Autodesk Inventor part; units mm, degrees
(part 2 of 2)
sketch "Skizze22" plane through (45, 45.75, 168) normal (0, 1, 0) x (1, 0, 0)
  line L0 (15, 0) -> (0, 0) projected
  line L1 (15, 168) -> (15, 0) projected
  line L2 (0, 168) -> (15, 168) projected
  line L3 (-105, 0) -> (-105, 168) projected
  line L4 (-105, 168) -> (-90, 168) projected
  line L5 (-90, 0) -> (-105, 0) projected
  circle A0 centre (-97.5, 7.5) radius 1.35 projected
  circle A1 centre (-97.5, 7.5) radius 1.7
  circle A2 centre (7.5, 7.5) radius 1.7
  circle A3 centre (7.5, 142.5) radius 1.7
  circle A4 centre (-97.5, 142.5) radius 1.7
  circle A5 centre (-97.5, 7.5) radius 1.35 construction
  line L6 (-97.5, 7.5) -> (-97.5, 142.5) construction
  line L7 (7.5, 142.5) -> (7.5, 7.5) construction
  circle A6 centre (7.5, 57.5) radius 1.7
  circle A7 centre (-97.5, 57.5) radius 1.7
  circle A8 centre (112.5, -130.5) radius 1.35
  circle A9 centre (112.5, -130.5) radius 1.7
  circle A10 centre (7.5, -130.5) radius 1.35
  circle A11 centre (7.5, -130.5) radius 1.7
  circle A12 centre (7.5, -25.5) radius 1.35
  circle A13 centre (7.5, -25.5) radius 1.7
  circle A14 centre (112.5, -25.5) radius 1.35
  circle A15 centre (112.5, -25.5) radius 1.7
  circle A16 centre (7.5, 7.5) radius 1.35
  circle A17 centre (7.5, 7.5) radius 1.7
  circle A18 centre (-97.5, 7.5) radius 1.35
  circle A19 centre (-97.5, 7.5) radius 1.7
  circle A20 centre (-97.5, 112.5) radius 1.35
  circle A21 centre (-97.5, 112.5) radius 1.7
  circle A22 centre (7.5, 112.5) radius 1.35
  circle A23 centre (7.5, 112.5) radius 1.7
  point P0 (-45, 168)
  point P1 (-97.5, 142.5)
  point P2 (-98.85, 7.5)
  point P3 (-98.85, 7.5)
  point P4 (7.5, 57.5)
  point P5 (60, 0)
  dimension "d104" = 7.5
  dimension "d105" = 7.5
  dimension "d106" = 25.5
  dimension "d107" = 7.5
  dimension "d108" = 7.5
  dimension "d109" = 25.5
  dimension "d110" = 7.5
  dimension "d111" = 7.5
  dimension "d113" = 3.4
  dimension "d114" = 3.4
  dimension "d115" = 3.4
  dimension "d129" = 3.4
  dimension "d130" = 135
  dimension "d131" = 50
  dimension "d132" = 50
  dimension "d133" = 3.4
  dimension "d134" = 3.4
  dimension "d165" = 3.4
  dimension "d166" = 3.4
  dimension "d167" = 3.4
  dimension "d168" = 3.4
  dimension "d169" = 3.4
  dimension "d170" = 3.4
  dimension "d171" = 3.4
  dimension "d172" = 3.4
  constraints: 22 centre point, 11 coincident, 4 end point, 2 point on line, 1 parallel
  measures "d104" distance from line of L0 point (7.5, 7.5)
  measures "d105" distance from line of L1 point (7.5, 7.5)
  measures "d106" distance from line of L2 point (7.5, 142.5)
  measures "d107" distance from line of L1 point (7.5, 142.5)
  measures "d108" distance from line of L3 point (-97.5, 142.5)
  measures "d109" distance from line of L4 point (-97.5, 142.5)
  measures "d110" distance from line of L3 point (-97.5, 7.5)
  measures "d111" distance from line of L5 point (-97.5, 7.5)
  measures "d113" diameter of A3
  measures "d114" diameter of A2
  measures "d115" diameter of A1
  measures "d129" diameter of A4
  measures "d130" distance of L7.start L7.end
  measures "d131" distance of point (7.5, 7.5) point (7.5, 57.5)
  measures "d132" distance of point (-97.5, 7.5) point (-97.5, 57.5)
  measures "d133" diameter of A6
  measures "d134" diameter of A7
  measures "d165" diameter of A15
  measures "d166" diameter of A13
  measures "d167" diameter of A11
  measures "d168" diameter of A9
  measures "d169" diameter of A23
  measures "d170" diameter of A21
  measures "d171" diameter of A19
  measures "d172" diameter of A17
extrude "Extrusion15" cut sketch "Skizze22" against normal blind 60 contours A0 | A1 | A2 | A3 | A4 | A6 | A7 | A16 | A20 | A21 | A22 | A23
ref_plane "Arbeitsebene1" through (45, 35.75, 168) normal (0, 1, 0) x (1, 0, 0)
sketch "Skizze23" plane through (45, 35.75, 168) normal (0, 1, 0) x (1, 0, 0)
  circle A0 centre (7.5, 7.5) radius 1.7 projected
  line L0 (4.65, 9.1454) -> (7.5, 10.7909)
  line L1 (7.5, 10.7909) -> (10.35, 9.1454)
  line L2 (10.35, 9.1454) -> (10.35, 5.8546)
  line L3 (10.35, 5.8546) -> (7.5, 4.2091)
  line L4 (7.5, 4.2091) -> (4.65, 5.8546)
  line L5 (4.65, 5.8546) -> (4.65, 9.1454)
  line L6 (0, 149.5) -> (0, 0) projected
  circle A1 centre (-97.5, 7.5) radius 1.7 projected
  circle A2 centre (7.5, 142.5) radius 1.7 projected
  line L7 (-100.35, 9.1454) -> (-97.5, 10.7909)
  line L8 (-97.5, 10.7909) -> (-94.65, 9.1454)
  line L9 (-94.65, 9.1454) -> (-94.65, 5.8546)
  line L10 (-94.65, 5.8546) -> (-97.5, 4.2091)
  line L11 (-97.5, 4.2091) -> (-100.35, 5.8546)
  line L12 (-100.35, 5.8546) -> (-100.35, 9.1454)
  line L13 (15, 0) -> (0, 0)
  line L14 (15, 168) -> (15, 0)
  line L15 (0, 168) -> (15, 168)
  line L16 (-105, 0) -> (-105, 168)
  line L17 (-105, 168) -> (-90, 168)
  line L18 (-90, 0) -> (-105, 0)
  circle A3 centre (-97.5, 7.5) radius 1.35
  circle A4 centre (-97.5, 7.5) radius 1.7
  circle A5 centre (7.5, 7.5) radius 1.7
  circle A6 centre (7.5, 142.5) radius 1.7
  circle A7 centre (-97.5, 142.5) radius 1.7
  circle A8 centre (-97.5, 7.5) radius 1.35 construction
  line L19 (7.5, 142.5) -> (7.5, 7.5) construction
  line L20 (7.5, 4.2091) -> (15, 4.2091)
  line L21 (15, 0) -> (15, 168) projected
  line L22 (7.5, 10.7909) -> (15, 10.7909)
  line L23 (15, 4.2091) -> (15, 10.7909)
  line L24 (-97.5, 4.2091) -> (-105, 4.2091)
  line L25 (-105, 168) -> (-105, 0) projected
  line L26 (-97.5, 10.7909) -> (-105, 10.7909)
  line L27 (-105, 4.2091) -> (-105, 10.7909)
  line L28 (4.65, 144.1454) -> (7.5, 145.7909)
  line L29 (7.5, 145.7909) -> (10.35, 144.1454)
  line L30 (10.35, 144.1454) -> (10.35, 140.8546)
  line L31 (10.35, 140.8546) -> (7.5, 139.2091)
  line L32 (7.5, 139.2091) -> (4.65, 140.8546)
  line L33 (4.65, 140.8546) -> (4.65, 144.1454)
  line L34 (-100.35, 140.8546) -> (-100.35, 144.1454)
  line L35 (-100.35, 144.1454) -> (-97.5, 145.7909)
  line L36 (-97.5, 145.7909) -> (-94.65, 144.1454)
  line L37 (-94.65, 144.1454) -> (-94.65, 140.8546)
  line L38 (-94.65, 140.8546) -> (-97.5, 139.2091)
  line L39 (-97.5, 139.2091) -> (-100.35, 140.8546)
  circle A9 centre (7.5, 142.5) radius 1.7
  circle A10 centre (-97.5, 142.5) radius 1.35
  circle A11 centre (-97.5, 142.5) radius 1.35 construction
  circle A12 centre (-97.5, 142.5) radius 1.7
  line L40 (7.5, 139.2091) -> (15, 139.2091)
  line L41 (7.5, 145.7909) -> (15, 145.7909)
  line L42 (15, 139.2091) -> (15, 145.7909)
  line L43 (-97.5, 139.2091) -> (-105, 139.2091)
  line L44 (-97.5, 145.7909) -> (-105, 145.7909)
  line L45 (-105, 139.2091) -> (-105, 145.7909)
  line L46 (15, 0) -> (0, 0)
  line L47 (15, 168) -> (15, 0)
  line L48 (0, 168) -> (15, 168)
  line L49 (-105, 0) -> (-105, 168)
  line L50 (-105, 168) -> (-90, 168)
  line L51 (-90, 0) -> (-105, 0)
  circle A13 centre (-97.5, 7.5) radius 1.35
  circle A14 centre (-97.5, 7.5) radius 1.7
  circle A15 centre (7.5, 7.5) radius 1.7
  circle A16 centre (7.5, 142.5) radius 1.7
  circle A17 centre (-97.5, 142.5) radius 1.7
  circle A18 centre (-97.5, 7.5) radius 1.35 construction
  line L52 (-97.5, 7.5) -> (-97.5, 142.5) construction
  line L53 (7.5, 142.5) -> (7.5, 7.5) construction
  circle A19 centre (7.5, 57.5) radius 1.7
  circle A20 centre (-97.5, 57.5) radius 1.7
  circle A21 centre (-97.5, 112.5) radius 1.35
  circle A22 centre (-97.5, 112.5) radius 1.7
  circle A23 centre (-97.5, 7.5) radius 1.35
  circle A24 centre (-97.5, 7.5) radius 1.7
  circle A25 centre (7.5, 112.5) radius 1.35
  circle A26 centre (7.5, 112.5) radius 1.7
  circle A27 centre (7.5, 7.5) radius 1.35
  circle A28 centre (7.5, 7.5) radius 1.7
  circle A29 centre (7.5, 57.5) radius 1.7
  circle A30 centre (-97.5, 57.5) radius 1.7
  line L54 (4.65, 59.1454) -> (7.5, 60.7909)
  line L55 (7.5, 60.7909) -> (10.35, 59.1454)
  line L56 (10.35, 59.1454) -> (10.35, 55.8546)
  line L57 (10.35, 55.8546) -> (7.5, 54.2091)
  line L58 (7.5, 54.2091) -> (4.65, 55.8546)
  line L59 (4.65, 55.8546) -> (4.65, 59.1454)
  circle A31 centre (7.5, 57.5) radius 1.7
  line L60 (15, 54.2091) -> (15, 60.7909)
  line L61 (7.5, 54.2091) -> (15, 54.2091)
  line L62 (-97.5, 60.7909) -> (-94.65, 59.1454)
  line L63 (-94.65, 59.1454) -> (-94.65, 55.8546)
  line L64 (-100.35, 59.1454) -> (-97.5, 60.7909)
  line L65 (-94.65, 55.8546) -> (-97.5, 54.2091)
  line L66 (-100.35, 55.8546) -> (-100.35, 59.1454)
  line L67 (-97.5, 54.2091) -> (-100.35, 55.8546)
  line L68 (7.5, 60.7909) -> (15, 60.7909)
  line L69 (-97.5, 60.7909) -> (-105, 60.7909)
  circle A32 centre (-97.5, 57.5) radius 1.35
  circle A33 centre (-97.5, 57.5) radius 1.35 construction
  circle A34 centre (-97.5, 57.5) radius 1.7
  line L70 (-105, 54.2091) -> (-105, 60.7909)
  line L71 (-97.5, 54.2091) -> (-105, 54.2091)
  circle A35 centre (7.5, 112.5) radius 1.7
  circle A36 centre (-97.5, 112.5) radius 1.7
  line L72 (4.65, 114.1454) -> (7.5, 115.7909)
  line L73 (7.5, 115.7909) -> (10.35, 114.1454)
  line L74 (10.35, 114.1454) -> (10.35, 110.8546)
  line L75 (10.35, 110.8546) -> (7.5, 109.2091)
  line L76 (7.5, 109.2091) -> (4.65, 110.8546)
  line L77 (4.65, 110.8546) -> (4.65, 114.1454)
  circle A37 centre (7.5, 112.5) radius 1.7
  line L78 (15, 109.2091) -> (15, 115.7909)
  line L79 (7.5, 109.2091) -> (15, 109.2091)
  line L80 (-97.5, 115.7909) -> (-94.65, 114.1454)
  line L81 (-94.65, 114.1454) -> (-94.65, 110.8546)
  line L82 (-100.35, 114.1454) -> (-97.5, 115.7909)
  line L83 (-94.65, 110.8546) -> (-97.5, 109.2091)
  line L84 (-100.35, 110.8546) -> (-100.35, 114.1454)
  line L85 (-97.5, 109.2091) -> (-100.35, 110.8546)
  line L86 (7.5, 115.7909) -> (15, 115.7909)
  line L87 (-97.5, 115.7909) -> (-105, 115.7909)
  circle A38 centre (-97.5, 112.5) radius 1.35
  circle A39 centre (-97.5, 112.5) radius 1.35 construction
  circle A40 centre (-97.5, 112.5) radius 1.7
  line L88 (-105, 109.2091) -> (-105, 115.7909)
  line L89 (-97.5, 109.2091) -> (-105, 109.2091)
  point P0 (-45, 168)
  point P1 (-45, 168)
  point P2 (-97.5, 142.5)
  point P3 (-98.85, 7.5)
  point P4 (-98.85, 7.5)
  point P5 (-98.85, 142.5)
  point P6 (-98.85, 142.5)
  point P7 (-105, 10.7909)
  point P8 (7.5, 4.2091)
  point P9 (15, 4.2091)
  point P10 (15, 10.7909)
  point P11 (-45, 168)
  point P12 (-97.5, 142.5)
  point P13 (-98.85, 7.5)
  point P14 (-98.85, 7.5)
  point P15 (60, 0)
  point P16 (-98.85, 57.5)
  point P17 (-98.85, 57.5)
  point P18 (-98.85, 112.5)
  point P19 (-98.85, 112.5)
  point P20 (-105, 60.7909)
  point P21 (7.5, 54.2091)
  point P22 (15, 54.2091)
  point P23 (15, 60.7909)
  dimension "d119" = 5.7
  dimension "d120" = 5.7
  dimension "d135" = 7.5
  dimension "d136" = 7.5
  dimension "d137" = 25.5
  dimension "d138" = 7.5
  dimension "d139" = 7.5
  dimension "d140" = 25.5
  dimension "d141" = 7.5
  dimension "d142" = 7.5
  dimension "d143" = 3.4
  dimension "d144" = 3.4
  dimension "d145" = 3.4
  dimension "d146" = 3.4
  dimension "d147" = 135
  dimension "d156" = 5.7
  dimension "d157" = 5.7
  dimension "d158" = 3.4
  dimension "d159" = 3.4
  dimension "d173" = 7.5
  dimension "d174" = 7.5
  dimension "d175" = 25.5
  dimension "d176" = 7.5
  dimension "d177" = 7.5
  dimension "d178" = 25.5
  dimension "d179" = 7.5
  dimension "d180" = 7.5
  dimension "d181" = 3.4
  dimension "d182" = 3.4
  dimension "d183" = 3.4
  dimension "d184" = 3.4
  dimension "d185" = 135
  dimension "d186" = 50
  dimension "d187" = 50
  dimension "d188" = 3.4
  dimension "d189" = 3.4
  dimension "d190" = 3.4
  dimension "d191" = 3.4
  dimension "d192" = 3.4
  dimension "d193" = 3.4
  dimension "d194" = 3.4
  dimension "d195" = 3.4
  dimension "d196" = 5.7
  dimension "d197" = 5.7
  dimension "d198" = 3.4
  dimension "d199" = 3.4
  dimension "d200" = 3.4
  dimension "d201" = 3.4
  dimension "d202" = 5.7
  dimension "d203" = 5.7
  dimension "d204" = 3.4
  dimension "d205" = 3.4
  constraints: 174 end point, 38 centre point, 19 coincident, 10 perpendicular, 6 parallel, 6 point on line, 4 horizontal, 104 other
  measures "d119" distance between parallel lines of L2 L5
  measures "d120" distance between parallel lines of L9 L12
  measures "d135" distance from line of L13 point (7.5, 7.5)
  measures "d136" distance from line of L14 point (7.5, 7.5)
  measures "d137" distance from line of L15 point (7.5, 142.5)
  measures "d138" distance from line of L14 point (7.5, 142.5)
  measures "d139" distance from line of L16 point (-97.5, 142.5)
  measures "d140" distance from line of L17 point (-97.5, 142.5)
  measures "d141" distance from line of L16 point (-97.5, 7.5)
  measures "d142" distance from line of L18 point (-97.5, 7.5)
  measures "d143" diameter of A6
  measures "d144" diameter of A5
  measures "d145" diameter of A4
  measures "d146" diameter of A7
  measures "d147" distance of L19.start L19.end
  measures "d156" distance between parallel lines of L30 L33
  measures "d157" distance between parallel lines of L37 L34
  measures "d158" diameter of A9
  measures "d159" diameter of A12
  measures "d173" distance from line of L46 point (7.5, 7.5)
  measures "d174" distance from line of L47 point (7.5, 7.5)
  measures "d175" distance from line of L48 point (7.5, 142.5)
  measures "d176" distance from line of L47 point (7.5, 142.5)
  measures "d177" distance from line of L49 point (-97.5, 142.5)
  measures "d178" distance from line of L50 point (-97.5, 142.5)
  measures "d179" distance from line of L49 point (-97.5, 7.5)
  measures "d180" distance from line of L51 point (-97.5, 7.5)
  measures "d181" diameter of A16
  measures "d182" diameter of A15
  measures "d183" diameter of A14
  measures "d184" diameter of A17
  measures "d185" distance of L53.start L53.end
  measures "d186" distance of point (7.5, 7.5) point (7.5, 57.5)
  measures "d187" distance of point (-97.5, 7.5) point (-97.5, 57.5)
  measures "d188" diameter of A19
  measures "d189" diameter of A20
  measures "d190" diameter of A26
  measures "d191" diameter of A22
  measures "d192" diameter of A24
  measures "d193" diameter of A28
  measures "d194" diameter of A29
  measures "d195" diameter of A30
  measures "d196" distance between parallel lines of L56 L59
  measures "d197" distance between parallel lines of L63 L66
  measures "d198" diameter of A31
  measures "d199" diameter of A34
  measures "d200" diameter of A35
  measures "d201" diameter of A36
  measures "d202" distance between parallel lines of L74 L77
  measures "d203" distance between parallel lines of L81 L84
  measures "d204" diameter of A37
  measures "d205" diameter of A40
extrude "Extrusion16" cut sketch "Skizze23" against normal blind 2.6 contours A0 | L40 L31 L30 L29 L41 L14 | L79 L75 L74 L73 L86 L14 | L61 L57 L56 L55 L68 L14 | L0 L1 L2 L3 L4 L5 | L22 L14 L20 L3 L2 L1 | L58 L59 L54 L55 L56 L57 | L76 L77 L72 L73 L74 L75 | L32 L33 L28 L29 L30 L31 | A2 | L12 L11 L24 L16 L26 L7 | L7 L8 L9 L10 L11 L12 | L16 L44 L35 L34 L39 L43 | L16 L87 L82 L84 L85 L89 | L16 L69 L64 L66 L67 L71 | L67 L66 L64 L62 L63 L65 | L85 L84 L82 L80 L81 L83 | L39 L34 L35 L36 L37 L38 | A19 | A27
sketch "Skizze24" plane through (60, -60.989, 0) normal (1, 0, 0) x (0, 0, -1)
  line L0 (-163.7909, 96.739) -> (-163.7909, 94.139) construction
  line L1 (-163.7909, 94.139) -> (-157.2091, 96.739) construction
  line L2 (-157.2091, 96.739) -> (-163.7909, 96.739) construction
  line L3 (-157.2091, 96.739) -> (-157.2091, 94.139) construction
  line L4 (-163.7909, 96.739) -> (-157.2091, 94.139) construction
  line L5 (-163.7909, 94.139) -> (-157.2091, 94.139) construction
  line L6 (-113.7909, 94.139) -> (-107.2091, 96.739) construction
  line L7 (-107.2091, 96.739) -> (-113.7909, 96.739) construction
  line L8 (-113.7909, 96.739) -> (-107.2091, 94.139) construction
  line L9 (-28.7909, 94.139) -> (-28.7909, 96.739) construction
  line L10 (-28.7909, 96.739) -> (-22.2091, 96.739) construction
  line L11 (-28.7909, 94.139) -> (-22.2091, 96.739) construction
  line L12 (-22.2091, 96.739) -> (-28.7909, 96.739) construction
  line L13 (-23.8546, 94.139) -> (-22.2091, 94.139) construction
  line L14 (-28.7909, 96.739) -> (-22.2091, 94.139) construction
  circle A0 centre (-25.5, 95.439) radius 0.8
  circle A1 centre (-110.5, 95.439) radius 0.8
  circle A2 centre (-160.5, 95.439) radius 0.8
  line L15 (-112.1454, 94.139) -> (-113.7909, 94.139) projected
  line L16 (-58.7909, 94.139) -> (-57.1454, 94.139) projected
  line L17 (-58.7909, 94.139) -> (-52.2091, 96.739) construction
  line L18 (-52.2091, 96.739) -> (-58.7909, 96.739) construction
  line L19 (-58.7909, 96.739) -> (-52.2091, 94.139) construction
  circle A3 centre (-55.5, 95.439) radius 0.8
  point P0 (0, 60.989)
  point P1 (-96.2909, 94.139)
  point P2 (-89.7091, 94.139)
  point P3 (-58.7909, 94.139)
  dimension "d_Mutterwechsel" = 1.6
  dimension "d161" = 1.6
  dimension "d162" = 1.6
  dimension "d206" = 1.6
  constraints: 24 end point, 4 centre point, 4 midpoint, 2 equal length, 1 horizontal
  measures "d_Mutterwechsel" diameter of A0
  measures "d161" diameter of A2
  measures "d162" diameter of A1
  measures "d206" diameter of A3
extrude "Extrusion17" cut sketch "Skizze24" against normal through all
sketch "Sketch25" plane through (60, -60.989, 0) normal (1, 0, 0) x (0, 0, -1)
  circle A0 centre (-84, 62.114) radius 35.025
  line L0 (-168, 106.739) -> (-168, 17.489) construction
  line L1 (0, 0) -> (-3, 0) construction
  line L2 (-168, 106.739) -> (0, 0) construction
  line L3 (0, 0) -> (-168, 0) construction
  line L4 (-168, 0) -> (0, 106.739) construction
  line L5 (-84, 53.3695) -> (-84, 106.739) construction
  line L6 (0, 106.739) -> (-168, 106.739) construction
  line L7 (-59.5, 62.114) -> (-84, 62.114) construction
  circle A1 centre (-84, 62.114) radius 11.25
  point P0 (0, 60.989)
  point P1 (0, 60.989)
  dimension "d208" = 70.05
  dimension "d209" = 22.5
  constraints: 10 end point, 2 centre point, 2 coincident, 2 midpoint, 1 collinear, 1 horizontal, 1 perpendicular, 1 point on line
  measures "d208" diameter of A0
  measures "d209" diameter of A1
extrude "Extrusion18" cut sketch "Sketch25" against normal through all contours A1
sketch "Sketch26" plane through (60, -60.989, 0) normal (1, 0, 0) x (0, 0, -1)
  circle A0 centre (-84, 62.114) radius 35.025
  line L0 (-84, 53.3695) -> (-84, 106.739) construction
  line L1 (-59.5, 62.114) -> (-84, 62.114) construction
  circle A1 centre (-84, 62.114) radius 11.25
  point P0 (0, 60.989)
  dimension "d212" = 70.05
  dimension "d213" = 22.5
  constraints: 4 end point, 2 centre point, 2 coincident, 1 horizontal, 1 point on line
  measures "d212" diameter of A0
  measures "d213" diameter of A1
extrude "Extrusion19" cut sketch "Sketch26" against normal blind 13
mirror "Mirror1" about plane through (0, 0, 0) normal (1, 0, 0) of "Extrusion19"
sketch "Sketch27" plane through (60, -60.989, 0) normal (1, 0, 0) x (0, 0, -1)
  circle A0 centre (-61.5494, 84.5646) radius 3
  circle A1 centre (-61.5494, 84.5646) radius 5
  circle A2 centre (-84, 62.114) radius 11.25
  circle A3 centre (-84, 62.114) radius 11.25
  circle A4 centre (-106.4506, 84.5646) radius 5
  circle A5 centre (-106.4506, 39.6633) radius 5
  circle A6 centre (-61.5494, 39.6633) radius 5
  circle A7 centre (-84, 62.114) radius 11.25 projected
  point P0 (0, 60.989)
  dimension "d218" = 10
  dimension "d219" = 360
  constraints: 7 centre point, 3 coincident, 9 other
  measures "d218" diameter of A1
extrude "Extrusion20" cut sketch "Sketch27" against normal through all contours A0 | A1 | A4 | A5 | A6
chamfer "Chamfer1" distance 1.5 angle 45 8 edges at (45, 23.5756, 66.5494) (45, 23.5756, 111.4506) (45, -21.3256, 66.5494) (45, -21.3256, 111.4506) (-45, -21.3256, 111.4506) (-45, -21.3256, 66.5494) (-45, 23.5756, 111.4506) (-45, 23.5756, 66.5494)
sketch "Sketch28" plane through (60, -60.989, 0) normal (1, 0, 0) x (0, 0, -1)
  line L0 (49.8957, 23.75) -> (46.8957, 23.75)
  line L1 (46.8957, 23.75) -> (46.8957, 97.75)
  line L2 (46.8957, 97.75) -> (49.8957, 97.75)
  line L3 (49.8957, 97.75) -> (49.8957, 23.75)
  circle A0 centre (48.3957, 60.75) radius 11.25
  line L4 (49.8957, 23.75) -> (46.8957, 97.75) construction
  line L5 (46.8957, 23.75) -> (49.8957, 97.75) construction
  line L6 (48.3957, 60.75) -> (46.8957, 60.75)
  line L7 (48.3957, 60.75) -> (49.8957, 60.75)
  line L8 (65.5966, 27.9571) -> (28.5966, 92.0429)
  line L9 (31.1947, 93.5429) -> (68.1947, 29.4571)
  line L10 (28.5966, 92.0429) -> (31.1947, 93.5429)
  line L11 (68.1947, 29.4571) -> (65.5966, 27.9571)
  line L12 (79.6886, 40.951) -> (15.6027, 77.951)
  line L13 (17.1027, 80.549) -> (81.1886, 43.549)
  line L14 (15.6027, 77.951) -> (17.1027, 80.549)
  line L15 (81.1886, 43.549) -> (79.6886, 40.951)
  line L16 (85.3957, 59.25) -> (11.3957, 59.25)
  line L17 (11.3957, 62.25) -> (85.3957, 62.25)
  line L18 (11.3957, 59.25) -> (11.3957, 62.25)
  line L19 (85.3957, 62.25) -> (85.3957, 59.25)
  line L20 (81.1886, 77.951) -> (17.1027, 40.951)
  line L21 (15.6027, 43.549) -> (79.6886, 80.549)
  line L22 (17.1027, 40.951) -> (15.6027, 43.549)
  line L23 (79.6886, 80.549) -> (81.1886, 77.951)
  line L24 (68.1947, 92.0429) -> (31.1947, 27.9571)
  line L25 (28.5966, 29.4571) -> (65.5966, 93.5429)
  line L26 (31.1947, 27.9571) -> (28.5966, 29.4571)
  line L27 (65.5966, 93.5429) -> (68.1947, 92.0429)
  line L28 (49.8957, 97.75) -> (49.8957, 23.75)
  line L29 (46.8957, 23.75) -> (46.8957, 97.75)
  line L30 (49.8957, 23.75) -> (46.8957, 23.75)
  line L31 (46.8957, 97.75) -> (49.8957, 97.75)
  line L32 (31.1947, 93.5429) -> (68.1947, 29.4571)
  line L33 (65.5966, 27.9571) -> (28.5966, 92.0429)
  line L34 (68.1947, 29.4571) -> (65.5966, 27.9571)
  line L35 (28.5966, 92.0429) -> (31.1947, 93.5429)
  line L36 (17.1027, 80.549) -> (81.1886, 43.549)
  line L37 (79.6886, 40.951) -> (15.6027, 77.951)
  line L38 (81.1886, 43.549) -> (79.6886, 40.951)
  line L39 (15.6027, 77.951) -> (17.1027, 80.549)
  line L40 (11.3957, 62.25) -> (85.3957, 62.25)
  line L41 (85.3957, 59.25) -> (11.3957, 59.25)
  line L42 (85.3957, 62.25) -> (85.3957, 59.25)
  line L43 (11.3957, 59.25) -> (11.3957, 62.25)
  line L44 (15.6027, 43.549) -> (79.6886, 80.549)
  line L45 (81.1886, 77.951) -> (17.1027, 40.951)
  line L46 (79.6886, 80.549) -> (81.1886, 77.951)
  line L47 (17.1027, 40.951) -> (15.6027, 43.549)
  line L48 (28.5966, 29.4571) -> (65.5966, 93.5429)
  line L49 (68.1947, 92.0429) -> (31.1947, 27.9571)
  line L50 (65.5966, 93.5429) -> (68.1947, 92.0429)
  line L51 (31.1947, 27.9571) -> (28.5966, 29.4571)
  circle A1 centre (48.3957, 60.75) radius 37.0304
  line L52 (227.9278, 109.8072) -> (175.6019, 162.1331)
  line L53 (177.7232, 164.2544) -> (230.0491, 111.9285)
  line L54 (230.0491, 111.9285) -> (227.9278, 109.8072)
  line L55 (175.6019, 162.1331) -> (177.7232, 164.2544)
  circle A2 centre (-84, 62.114) radius 11.25 projected
  line L56 (-56.7764, 37.0117) -> (-58.8977, 34.8904)
  line L57 (-58.8977, 34.8904) -> (-111.2236, 87.2163)
  line L58 (-109.1023, 89.3376) -> (-56.7764, 37.0117)
  line L59 (-111.2236, 87.2163) -> (-109.1023, 89.3376)
  line L60 (-47.8725, 53.9866) -> (-48.649, 51.0888)
  line L61 (-120.1275, 70.2414) -> (-119.351, 73.1392)
  line L62 (-119.351, 73.1392) -> (-47.8725, 53.9866)
  line L63 (-48.649, 51.0888) -> (-120.1275, 70.2414)
  line L64 (-48.649, 73.1392) -> (-47.8725, 70.2414)
  line L65 (-119.351, 51.0888) -> (-120.1275, 53.9866)
  line L66 (-120.1275, 53.9866) -> (-48.649, 73.1392)
  line L67 (-47.8725, 70.2414) -> (-119.351, 51.0888)
  line L68 (-58.8977, 89.3376) -> (-56.7764, 87.2163)
  line L69 (-109.1023, 34.8904) -> (-111.2236, 37.0117)
  line L70 (-111.2236, 37.0117) -> (-58.8977, 89.3376)
  line L71 (-56.7764, 87.2163) -> (-109.1023, 34.8904)
  line L72 (-75.8726, 98.2415) -> (-72.9748, 97.465)
  line L73 (-92.1274, 25.9865) -> (-95.0252, 26.763)
  line L74 (-95.0252, 26.763) -> (-75.8726, 98.2415)
  line L75 (-72.9748, 97.465) -> (-92.1274, 25.9865)
  line L76 (-95.0252, 97.465) -> (-92.1274, 98.2415)
  line L77 (-72.9748, 26.763) -> (-75.8726, 25.9865)
  line L78 (-75.8726, 25.9865) -> (-95.0252, 97.465)
  line L79 (-92.1274, 98.2415) -> (-72.9748, 26.763)
  line L80 (-111.2236, 87.2163) -> (-109.1023, 89.3376)
  line L81 (-56.7764, 37.0117) -> (-58.8977, 34.8904)
  line L82 (-58.8977, 34.8904) -> (-111.2236, 87.2163)
  line L83 (-109.1023, 89.3376) -> (-56.7764, 37.0117)
  line L84 (-120.1275, 70.2414) -> (-119.351, 73.1392)
  line L85 (-47.8725, 53.9866) -> (-48.649, 51.0888)
  line L86 (-48.649, 51.0888) -> (-120.1275, 70.2414)
  line L87 (-119.351, 73.1392) -> (-47.8725, 53.9866)
  line L88 (-119.351, 51.0888) -> (-120.1275, 53.9866)
  line L89 (-48.649, 73.1392) -> (-47.8725, 70.2414)
  line L90 (-47.8725, 70.2414) -> (-119.351, 51.0888)
  line L91 (-120.1275, 53.9866) -> (-48.649, 73.1392)
  line L92 (-109.1023, 34.8904) -> (-111.2236, 37.0117)
  line L93 (-58.8977, 89.3376) -> (-56.7764, 87.2163)
  line L94 (-56.7764, 87.2163) -> (-109.1023, 34.8904)
  line L95 (-111.2236, 37.0117) -> (-58.8977, 89.3376)
  line L96 (-92.1274, 25.9865) -> (-95.0252, 26.763)
  line L97 (-75.8726, 98.2415) -> (-72.9748, 97.465)
  line L98 (-72.9748, 97.465) -> (-92.1274, 25.9865)
  line L99 (-95.0252, 26.763) -> (-75.8726, 98.2415)
  line L100 (-72.9748, 26.763) -> (-75.8726, 25.9865)
  line L101 (-95.0252, 97.465) -> (-92.1274, 98.2415)
  line L102 (-92.1274, 98.2415) -> (-72.9748, 26.763)
  line L103 (-75.8726, 25.9865) -> (-95.0252, 97.465)
  point P0 (0, 60.989)
  point P1 (48.3957, 110.5)
  point P2 (47.0966, 60)
  point P3 (49.6947, 61.5)
  point P4 (47.6457, 59.451)
  point P5 (49.1457, 62.049)
  point P6 (48.3957, 59.25)
  point P7 (48.3957, 62.25)
  point P8 (49.1457, 59.451)
  point P9 (47.6457, 62.049)
  point P10 (49.6947, 60)
  point P11 (47.0966, 61.5)
  point P12 (49.8957, 60.75)
  point P13 (46.8957, 60.75)
  point P14 (49.6947, 61.5)
  point P15 (47.0966, 60)
  point P16 (49.1457, 62.049)
  point P17 (47.6457, 59.451)
  point P18 (48.3957, 62.25)
  point P19 (48.3957, 59.25)
  point P20 (47.6457, 62.049)
  point P21 (49.1457, 59.451)
  point P22 (47.0966, 61.5)
  point P23 (49.6947, 60)
  point P24 (202.8255, 137.0308)
  point P25 (203.8861, 138.0915)
  point P26 (201.7648, 135.9702)
  point P27 (-82.9393, 63.1746)
  point P28 (-84, 62.114)
  point P29 (-85.0607, 61.0533)
  point P30 (-83.6118, 63.5629)
  point P31 (-84, 62.114)
  point P32 (-84.3882, 60.6651)
  point P33 (-84.3882, 63.5629)
  point P34 (-84, 62.114)
  point P35 (-83.6118, 60.6651)
  point P36 (-85.0607, 63.1746)
  point P37 (-84, 62.114)
  point P38 (-82.9393, 61.0533)
  point P39 (-85.4489, 62.5022)
  point P40 (-84, 62.114)
  point P41 (-82.5511, 61.7257)
  point P42 (-85.4489, 61.7257)
  point P43 (-84, 62.114)
  point P44 (-82.5511, 62.5022)
  point P45 (-85.0607, 61.0533)
  point P46 (-84, 62.114)
  point P47 (-82.9393, 63.1746)
  point P48 (-84.3882, 60.6651)
  point P49 (-84, 62.114)
  point P50 (-83.6118, 63.5629)
  point P51 (-83.6118, 60.6651)
  point P52 (-84, 62.114)
  point P53 (-84.3882, 63.5629)
  point P54 (-82.9393, 61.0533)
  point P55 (-84, 62.114)
  point P56 (-85.0607, 63.1746)
  point P57 (-82.5511, 61.7257)
  point P58 (-84, 62.114)
  point P59 (-85.4489, 62.5022)
  point P60 (-82.5511, 62.5022)
  point P61 (-84, 62.114)
  point P62 (-85.4489, 61.7257)
  point P63 (-78.2044, 62.114)
  point P64 (-81.8787, 64.2353)
  point P65 (-84, 67.9095)
  point P66 (-86.1213, 64.2353)
  point P67 (-89.7956, 62.114)
  point P68 (-86.1213, 59.9927)
  point P69 (-84, 56.3184)
  point P70 (-81.8787, 59.9927)
  dimension "d25" = 10
  dimension "d28" = 10
  dimension "d227" = 3
  dimension "d228" = 74
  dimension "d229" = 360
  dimension "d248" = 360
  constraints: 208 end point, 15 coincident, 8 midpoint, 4 parallel, 2 perpendicular, 1 centre point, 279 other
  measures "d227" distance of L2.start L2.end
  measures "d228" distance of L0.end L2.start
extrude "Extrusion21" cut sketch "Sketch28" against normal blind 13 contours L67 L62 L71 L66 A2 | A2 L66 L64 L67 | L62 L60 L63 A2 | A2 L63 L58 L67 L62 | L67 L58 L71 L62 | L71 L62 L75 L66 | L71 L58 L75 L62 | L67 L79 L71 L58 | L58 L63 L79 L67 | L75 L62 L79 L66 | L66 L79 L70 L75 | L75 L58 L79 L62 | L71 L79 L75 L58 | L79 L63 L75 L67 | L67 L75 L71 L79 | L79 L57 L75 L63 | L75 L70 L79 L74 A2 | A2 L74 L72 L75 | L79 L62 L58 L66 | L66 L58 L70 L79 | L79 L58 L62 | L75 L79 L58 | L71 L75 L79 | L75 L63 L71 L67 | L67 L71 L75 | L79 L77 L78 A2 | A2 L78 L75 L57 L79 | L75 L57 L71 L63 | L70 L58 L74 L79 | L66 L62 L70 L58 | L58 L62 L66 | L58 L79 L75 L71 L67 L63 L57 L78 L74 L70 L66 L62 | L71 L63 L67 | L75 L78 L71 L57 | L71 L57 L67 L63 | L79 L74 L58 L78 A2 | A2 L78 L76 L79 | L70 L62 L74 L58 | L66 L70 L62 | L67 L57 L63 | L75 L73 L74 A2 | A2 L74 L71 L78 L75 | L71 L78 L67 L57 | L74 L62 L78 L58 | L70 L66 L74 L62 | L70 L74 L66 | L63 L78 L57 | L57 L67 L78 L63 | L71 L74 L67 L78 | L74 L66 L78 L62 | L74 L70 L78 L66 | L74 L78 L70 | L78 L63 L74 L57 | L57 L74 L78 | L78 L67 L74 L63 | L78 L66 L57 L62 | L78 L70 L57 L66 | L78 L74 L57 L70 | L74 L63 L70 L57 | L74 L67 L70 L63 | L62 L57 L66 L63 A2 | A2 L63 L61 L62 | L57 L70 L63 L66 | L70 L67 A2 L66 L63 | L67 L65 L66 A2
mirror "Mirror2" about plane through (0, 0, 0) normal (1, 0, 0) of "Extrusion21"
sketch "Sketch29" plane through (-60, -60.989, 0) normal (-1, 0, 0) x (0, 0, 1)
  circle A0 centre (84, 62.114) radius 11.25 projected
  circle A1 centre (114, 62.114) radius 6
  circle A2 centre (54, 62.114) radius 6
  point P0 (0, 60.989)
  dimension "d" = 12
  dimension "d251" = 12
  dimension "d252" = 30
  dimension "d253" = 30
  constraints: 2 centre point, 1 coincident
  measures "d" diameter of A1
  measures "d251" diameter of A2
  measures "d252" distance of point (84, 62.114) A1.centre
  measures "d253" distance of point (84, 62.114) A2.centre
extrude "Extrusion22" cut sketch "Sketch29" against normal through all contours A1 | A2
sketch "Sketch30" plane through (60, -60.989, 0) normal (1, 0, 0) x (0, 0, -1)
  line L0 (-120.1275, 70.2414) -> (-119.351, 73.1392) projected
  line L1 (-47.8725, 53.9866) -> (-49.8113, 54.506) projected
  line L2 (-120.1275, 70.2414) -> (-47.8725, 53.9866)
  line L3 (-120.1275, 53.9866) -> (-118.1887, 54.506) projected
  line L4 (-47.8725, 70.2414) -> (-48.649, 73.1392) projected
  line L5 (-120.1275, 53.9866) -> (-47.8725, 70.2414)
  point P0 (0, 60.989)
  constraints: 4 end point
sketch "Sketch31" plane through (-60, -60.989, 168) normal (0, -1, 0) x (1, 0, 0)
  line L0 (0, 0) -> (15, 0) projected
  line L1 (120, 0) -> (120, -168) projected
  line L2 (0, 0) -> (120, 0)
  line L3 (120, 0) -> (120, -168)
  line L4 (120, -168) -> (0, -168)
  line L5 (0, -168) -> (0, 0)
  line L6 (105, -168) -> (105, -165) projected
  line L7 (15, 0) -> (15, -8.5) projected
  line L8 (105, -168) -> (15, -168)
  line L9 (15, -168) -> (15, 0)
  line L10 (15, 0) -> (105, 0)
  line L11 (105, 0) -> (105, -168)
  point P0 (60, -168)
  constraints: 16 end point, 4 parallel, 2 horizontal, 2 perpendicular
extrude "Extrusion23" [suppressed]
